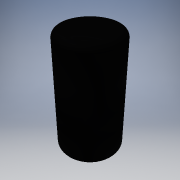
# Autodesk Inventor part: 1RBLK_TactileCap
Saved by Autodesk Inventor 2016 (Build 200138000, 138)
## iProperties
Created: 2016-09-23
Part Number: 1RBLK_TactileCap
Material: Generic
Document SubType Name: Modeling
Designer: jfixelle
Density: 1 g/cm^3
Appearance: Black
Author: jfixelle
Autodesk Inventor part; units mm, degrees
ref_plane "YZ Plane" through (0, 0, 0) normal (1, 0, 0) x (0, 1, 0)
ref_plane "XZ Plane" through (0, 0, 0) normal (0, 1, 0) x (-1, 0, 0)
ref_plane "XY Plane" through (0, 0, 0) normal (0, 0, 1) x (1, 0, 0)
sketch "Sketch1" plane through (0, 0, 0) normal (0, 1, 0) x (-1, 0, 0)
  circle A0 centre (0, 0) radius 2.54
  dimension "d0" = 5.08
  constraints: 1 centre point, 1 coincident
  measures "d0" diameter of A0
extrude "Extrusion1" add sketch "Sketch1" along normal blind 9.09
chamfer "Chamfer1" distance 9.09 angle 1 1 edges at (2.54, 9.09, 0) measured on face at (-2.5071, 3.03, -0.4074)
fillet "Fillet1" radius 0.5 1 edges at (2.3818, 9.09, 0)
sketch "Sketch2" plane through (0, 0, 0) normal (0, -1, 0) x (1, 0, 0)
  line L0 (1.4, -1.4) -> (-1.4, -1.4)
  line L1 (-1.4, -1.4) -> (-1.4, 1.4)
  line L2 (-1.4, 1.4) -> (1.4, 1.4)
  line L3 (1.4, 1.4) -> (1.4, -1.4)
  point P0 (0, 0)
  dimension "d7" = 2.8
  dimension "d8" = 1.4
  dimension "d9" = 2.8
  dimension "d10" = 1.4
  constraints: 8 end point, 2 parallel, 1 horizontal, 1 perpendicular
  measures "d7" distance of L0.start L0.end
  measures "d8" distance from line of point (0, 0) L1
  measures "d9" distance of L0.end L1.end
  measures "d10" distance from line of point (0, 0) L0
extrude "Extrusion2" cut sketch "Sketch2" against normal blind 2.95
body "Solid1"
